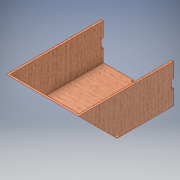
# Autodesk Inventor part: OpticalDeviceMirrorPart
Saved by Autodesk Inventor 2017 (Build 210142000, 142)
## iProperties
Created: 2019-04-02
Part Number: OpticalDeviceMirrorPart
Material: Generic
Document SubType Name: Modeling
Designer: Sharat
Density: 1 g/cm^3
Appearance: Red Oak - Natural Low Gloss
Author: Sharat
Autodesk Inventor part; units mm, degrees
ref_plane "YZ Plane" through (0, 0, 0) normal (1, 0, 0) x (0, 1, 0)
ref_plane "XZ Plane" through (0, 0, 0) normal (0, 1, 0) x (-1, 0, 0)
ref_plane "XY Plane" through (0, 0, 0) normal (0, 0, 1) x (1, 0, 0)
sketch "Sketch1" plane through (0, 0, 0) normal (0, 1, 0) x (-1, 0, 0)
  line L0 (0, 0) -> (170, 0)
  line L1 (170, 0) -> (170, -132.9)
  line L2 (0, -132.9) -> (0, 0)
  line L3 (170, -132.9) -> (95, -132.9)
  line L4 (75, -132.9) -> (0, -132.9)
  line L5 (95, -132.9) -> (95, -127.9)
  line L6 (95, -127.9) -> (75, -127.9)
  line L7 (75, -127.9) -> (75, -132.9)
  dimension "d0" = 132.9
  dimension "d22" = 170
  dimension "d23" = 75
  dimension "d24" = 75
  dimension "d41" = 5
  dimension "d42" = 5
  dimension "d43" = 75
  dimension "d44" = 20
  constraints: 16 end point, 3 perpendicular, 2 horizontal, 1 parallel, 1 point on line, 1 vertical
  measures "d0" distance of L0.end L1.end
  measures "d22" distance of L0.start L0.end
  measures "d23" distance of L1.end L3.end
  measures "d24" distance of L4.start L2.start
  measures "d41" distance of L6.end L4.start
  measures "d42" distance of L3.end L5.end
  measures "d43" distance between parallel lines of L2 L7
  measures "d44" distance of L5.end L6.end
extrude "Extrusion1" add sketch "Sketch1" along normal blind 4.7625
sketch "Sketch2" plane through (0, 4.7625, 0) normal (0, 1, 0) x (1, 0, 0)
  line L0 (-170, 0) -> (0, 0) projected
  line L1 (0, 132.9) -> (-170, 132.9) projected
  line L2 (-170, 0) -> (-170, 132.9)
  line L3 (-170, 132.9) -> (-165.2375, 132.9)
  line L4 (-165.2375, 132.9) -> (-165.2375, 0)
  line L5 (-170, 0) -> (-165.2375, 0)
  line L6 (0, 0) -> (-4.7625, 0)
  line L7 (-4.7625, 0) -> (-4.7625, 132.9)
  line L8 (-4.7625, 132.9) -> (0, 132.9)
  line L9 (0, 0) -> (0, 132.9) projected
  line L10 (0, 132.9) -> (0, 0)
  dimension "d4" = 4.7625
  dimension "d5" = 4.7625
  constraints: 16 end point, 4 perpendicular, 4 point on line, 2 vertical
  measures "d4" distance of L1.end L3.end
  measures "d5" distance of L0.end L6.end
extrude "Extrusion2" add sketch "Sketch2" along normal blind 85.2375 contours L7 L1 L9 L0
sketch "Sketch3" plane through (0, 4.7625, 0) normal (0, 1, 0) x (1, 0, 0)
  point P0 (0, 0)
sketch "Sketch4" plane through (-170, 0, -132.9) normal (-1, 0, 0) x (0, 0, 1)
  line L0 (132.9, 4.7625) -> (217.7528, 89.6153)
  line L1 (0, 4.7625) -> (132.9, 4.7625) projected
  line L2 (132.9, 0) -> (132.9, 4.7625) projected
  line L3 (0, 0) -> (132.9, 0) projected
  line L4 (132.9, 0) -> (220.1341, 87.2341)
  line L5 (220.1341, 87.2341) -> (217.7528, 89.6153)
  line L6 (132.9, 4.7625) -> (132.9, 0)
  dimension "d8" = 120
  dimension "d9" = 45
  constraints: 8 end point, 2 coincident, 2 perpendicular, 1 parallel
  measures "d8" distance of L0.start L0.end
  measures "d9" angle of L1 L0
sketch "Sketch5" plane through (0, 0, 0) normal (1, 0, 0) x (0, 0, -1)
  line L0 (0, 0) -> (0, 90) projected
  line L1 (0, 90) -> (-90, 90)
  line L2 (132.9, 0) -> (0, 0) projected
  line L3 (-90, 90) -> (0, 0)
  line L4 (0, 0) -> (0, 90)
  dimension "d11" = 45
  constraints: 6 end point, 1 horizontal, 1 vertical
  measures "d11" angle of L2 L3
extrude "Extrusion3" add sketch "Sketch5" against normal blind 105.2375
sketch "Sketch6" plane through (-105.2375, 0, 0) normal (-1, 0, 0) x (0, 0, 1)
  line L0 (0, 0) -> (0, 4.7625) projected
  line L1 (0, 4.7625) -> (0, 90)
  line L2 (-132.9, 90) -> (90, 90) projected
  line L3 (0, 90) -> (85.2375, 90)
  line L4 (85.2375, 90) -> (0, 4.7625)
  line L5 (0, 0) -> (90, 90) projected
  constraints: 6 end point, 2 point on line, 1 parallel, 1 vertical
extrude "Extrusion4" cut sketch "Sketch6" against normal blind 100.475 contours L1 L2 L4
sketch "Sketch7" plane through (-105.2375, 0, 0) normal (-1, 0, 0) x (0, 0, 1)
  line L0 (0, 4.7625) -> (0, 0)
  line L1 (0, 0) -> (90, 90)
  line L2 (85.2375, 90) -> (0, 4.7625) projected
  line L3 (90, 90) -> (85.2375, 90)
  line L4 (85.2375, 90) -> (0, 4.7625)
  constraints: 8 end point, 1 collinear, 1 perpendicular, 1 vertical
extrude "Extrusion5" add sketch "Sketch7" along normal blind 64.75
extrude "Extrusion6" add sketch "Sketch2" along normal blind 85.2375 contours L2 L1 L4 L0
sketch "Sketch8" plane through (-170, 0, -132.9) normal (-1, 0, 0) x (0, 0, 1)
  line L0 (0, 90) -> (222.9, 90) projected
  line L1 (132.9, 90) -> (218.1375, 90)
  line L2 (218.1375, 90) -> (132.9, 4.7625) projected
  line L3 (218.1375, 90) -> (132.9, 4.7625)
  line L4 (132.9, 4.7625) -> (132.9, 90)
  point P0 (132.9, 0)
  constraints: 6 end point, 2 point on line, 1 collinear, 1 perpendicular
extrude "Extrusion7" add sketch "Sketch8" against normal blind 4.7625
sketch "Sketch9" plane through (0, 0, -132.9) normal (1, 0, 0) x (0, 0, -1)
  line L0 (0, 0) -> (0, 90) projected
  line L1 (-5, 55) -> (0, 55)
  line L2 (0, 55) -> (0, 35)
  line L3 (0, 35) -> (-5, 35)
  line L4 (-5, 35) -> (-5, 55)
  line L5 (0, 90) -> (-222.9, 90) projected
  line L6 (0, 0) -> (-132.9, 0) projected
  dimension "d28" = 5
  dimension "d29" = 20
  dimension "d30" = 35
  dimension "d31" = 35
  constraints: 8 end point, 2 parallel, 1 horizontal, 1 perpendicular, 1 point on line
  measures "d28" distance of L1.start L1.end
  measures "d29" distance of L3.end L1.start
  measures "d30" distance between parallel lines of L5 L1
  measures "d31" distance between parallel lines of L6 L3
extrude "Extrusion8" cut sketch "Sketch9" against normal blind 4.7625
sketch "Sketch10" plane through (-170, 0, -132.9) normal (-1, 0, 0) x (0, 0, 1)
  line L0 (0, 0) -> (0, 90) projected
  line L1 (0, 55) -> (5, 55)
  line L2 (5, 55) -> (5, 35)
  line L3 (5, 35) -> (0, 35)
  line L4 (0, 35) -> (0, 55)
  line L5 (0, 90) -> (218.1375, 90) projected
  line L6 (132.9, 0) -> (0, 0) projected
  dimension "d34" = 20
  dimension "d35" = 5
  dimension "d36" = 35
  dimension "d37" = 35
  constraints: 8 end point, 2 parallel, 1 horizontal, 1 perpendicular, 1 point on line
  measures "d34" distance of L1.end L2.end
  measures "d35" distance of L1.start L1.end
  measures "d36" distance between parallel lines of L5 L1
  measures "d37" distance between parallel lines of L6 L3
extrude "Extrusion9" cut sketch "Sketch10" against normal blind 4.7625
fillet "Fillet1" radius 1 4 edges at (-167.6188, 55, -127.9) (-167.6188, 35, -127.9) (-2.3813, 35, -127.9) (-2.3813, 55, -127.9)
body "Solid1"
